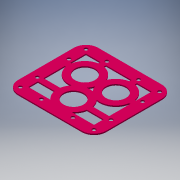
# Autodesk Inventor part: Base
Saved by Autodesk Inventor 2016 (Build 200138000, 138)
## iProperties
Created: 2015-03-29
Part Number: Base
Material: Generic
Document SubType Name: Modeling
Designer: Erin
Density: 1 g/cm^3
Appearance: Default
Author: Erin
Autodesk Inventor part; units mm, degrees
ref_plane "YZ Plane" through (0, 0, 0) normal (1, 0, 0) x (0, 1, 0)
ref_plane "XZ Plane" through (0, 0, 0) normal (0, 1, 0) x (-1, 0, 0)
ref_plane "XY Plane" through (0, 0, 0) normal (0, 0, 1) x (1, 0, 0)
sketch "Sketch1" plane through (0, 0, 0) normal (0, 0, 1) x (1, 0, 0)
  line L0 (-55, 50) -> (55, 50)
  line L1 (55, 50) -> (55, -50)
  line L2 (55, -50) -> (-55, -50)
  line L3 (-55, -50) -> (-55, 50)
  line L4 (41, 36) -> (-41, 36)
  line L5 (-41, 36) -> (-41, -36)
  line L6 (-41, -36) -> (41, -36)
  line L7 (41, -36) -> (41, 36)
  line L8 (0, 152.7233) -> (0, -72.1628) construction
  line L9 (-77.8847, 0) -> (88.8171, 0) construction
  line L10 (-55, 41) -> (55, 41) construction
  circle A0 centre (0, 41) radius 2.25
  circle A1 centre (-19.75, 41) radius 2.25
  circle A2 centre (19.75, 41) radius 2.25
  line L11 (-46, 50) -> (-46, -50) construction
  circle A3 centre (-46, 41) radius 2.25
  circle A4 centre (-46, 0) radius 2.25
  line L12 (-55, -41) -> (55, -41) construction
  circle A5 centre (-46, -41) radius 2.25
  circle A6 centre (-46, 19.75) radius 2.25
  circle A7 centre (-46, -19.75) radius 2.25
  line L13 (0, -20.5) -> (-19.3412, 13) construction
  line L14 (-19.3412, 13) -> (19.3412, 13) construction
  line L15 (19.3412, 13) -> (0, -20.5) construction
  circle A8 centre (19.3412, 13) radius 12.5
  circle A9 centre (-19.3412, 13) radius 12.5
  circle A10 centre (0, -20.5) radius 12.5
  circle A11 centre (-19.3412, 13) radius 20.5
  circle A12 centre (19.3412, 13) radius 20.5
  circle A13 centre (0, -20.5) radius 20.5
  line L16 (-22.8412, 30.0471) -> (-15.8412, 30.0471)
  line L17 (-15.8412, 30.0471) -> (-15.8412, 36)
  line L18 (-15.8412, 36) -> (-22.8412, 36)
  line L19 (-22.8412, 36) -> (-22.8412, 30.0471)
  line L20 (15.8412, 30.0471) -> (22.8412, 30.0471)
  line L21 (22.8412, 30.0471) -> (22.8412, 36)
  line L22 (22.8412, 36) -> (15.8412, 36)
  line L23 (15.8412, 36) -> (15.8412, 30.0471)
  line L24 (-35.3273, 16.5) -> (-41, 16.5)
  line L25 (-41, 16.5) -> (-41, 9.5)
  line L26 (-41, 9.5) -> (-35.3273, 9.5)
  line L27 (-35.3273, 9.5) -> (-35.3273, 16.5)
  line L28 (34.9738, 16.5) -> (41, 16.5)
  line L29 (41, 16.5) -> (41, 9.5)
  line L30 (41, 9.5) -> (34.9738, 9.5)
  line L31 (34.9738, 9.5) -> (34.9738, 16.5)
  line L32 (-3.5, -36.2367) -> (3.5, -36.2367)
  line L33 (3.5, -36.2367) -> (3.5, -36)
  line L34 (3.5, -36) -> (-3.5, -36)
  line L35 (-3.5, -36) -> (-3.5, -36.2367)
  line L36 (-16.3125, -17) -> (-41, -17)
  line L37 (-41, -17) -> (-41, -24)
  line L38 (-41, -24) -> (-16.3125, -24)
  line L39 (-16.3125, -24) -> (-16.3125, -17)
  line L40 (16.0929, -17) -> (41, -17)
  line L41 (41, -17) -> (41, -24)
  line L42 (41, -24) -> (16.0929, -24)
  line L43 (16.0929, -24) -> (16.0929, -17)
  point P0 (0, 0)
  point P1 (0, 50)
  point P2 (55, 0)
  point P3 (0, 1.8333)
  point P4 (-16.3125, -20.5)
  point P5 (16.0929, -20.5)
  point P6 (34.9738, 13)
  point P7 (-35.3273, 13)
  point P8 (-19.3412, 30.0471)
  point P9 (19.3412, 30.0471)
  point P10 (0, -36.2367)
  dimension "d0" = 110
  dimension "d1" = 100
  dimension "d2" = 14
  dimension "d5" = 9
  dimension "d6" = 4.5
  dimension "d7" = 4.5
  dimension "d8" = 4.5
  dimension "d9" = 22
  dimension "d10" = 22
  dimension "d11" = 9
  dimension "d12" = 4.5
  dimension "d13" = 4.5
  dimension "d14" = 9
  dimension "d15" = 4.5
  dimension "d31" = 4.5
  dimension "d32" = 4.5
  dimension "d33" = 22
  dimension "d34" = 22
  dimension "d53" = 23
  dimension "d54" = 25
  dimension "d55" = 25
  dimension "d56" = 25
  dimension "d65" = 8
  dimension "d66" = 8
  dimension "d67" = 8
  dimension "d68" = 7
  dimension "d69" = 7
  dimension "d70" = 7
  dimension "d71" = 7
  dimension "d72" = 7
  dimension "d73" = 7
  dimension "d74" = 7
  dimension "d75" = 38.6825
  constraints: 88 end point, 23 point on line, 19 parallel, 14 centre point, 13 perpendicular, 11 midpoint, 9 horizontal, 6 coincident, 5 horizontal alignment, 4 vertical alignment, 1 vertical, 10 other
  measures "d0" distance of L1.end L2.end
  measures "d1" distance of L0.end L1.end
  measures "d2" distance between parallel lines of L4 L0
  measures "d5" distance between parallel lines of L10 L0
  measures "d6" diameter of A0
  measures "d7" diameter of A1
  measures "d8" diameter of A2
  measures "d11" distance between parallel lines of L11 L3
  measures "d12" diameter of A3
  measures "d13" diameter of A4
  measures "d14" distance between parallel lines of L12 L2
  measures "d15" diameter of A5
  measures "d31" diameter of A6
  measures "d32" diameter of A7
  measures "d53" distance between parallel lines of L14 L4
  measures "d54" diameter of A8
  measures "d55" diameter of A9
  measures "d56" diameter of A10
  measures "d65" radial gap between concentric circles of A9 A11
  measures "d66" radial gap between concentric circles of A8 A12
  measures "d67" radial gap between concentric circles of A10 A13
  measures "d68" distance of L16.start L16.end
  measures "d69" distance of L20.start L20.end
  measures "d70" distance of L26.end L24.start
  measures "d71" distance of L30.end L28.start
  measures "d72" distance of L38.end L36.start
  measures "d73" distance of L42.end L40.start
  measures "d74" distance of L32.start L32.end
  measures "d75" distance of L13.end L14.end
extrude "Extrusion1" add sketch "Sketch1" along normal blind 1.5 contours L0 L1 L2 L3 | L21 A12 L23 L4 | L7 L30 A12 L28 | L21 L20 L23 A12 | A12 L28 L31 L30 A13 A11 L23 L20 L21 | A12 L30 L31 L28 | L17 A11 L19 L4 | L7 L42 A13 L40 | L17 L16 L19 A11 | A11 A12 A13 L26 L27 L24 L19 L16 L17 | A11 A12 | L40 L43 L42 A13 L6 L38 L39 L36 A11 A12 | A13 L42 L43 L40 | A12 A13 | L24 A11 L26 L5 | L24 L27 L26 A11 | A11 A13 | A13 L6 L35 L32 L33 | L33 L32 L35 L6 | L36 A13 L38 L5 | L36 L39 L38 A13 | A0 | A1 | A2 | A3 | A4 | A5 | A6 | A7
extrude "Extrusion2" cut sketch "Sketch1" along normal blind 10 contours A1 | A2
mirror "Mirror1" about plane through (0, 0, 0) normal (0, 1, 0) of "Extrusion2"
extrude "Extrusion3" cut sketch "Sketch1" along normal blind 10 contours A3 | A5 | A6 | A7
mirror "Mirror2" about plane through (0, 0, 0) normal (1, 0, 0) of "Extrusion3"
extrude "Extrusion7" cut sketch "Sketch1" along normal blind 10 contours L7 L28 A12 L21 L4 | L23 A12 A11 L17 L4 | L7 L40 A13 A12 L30 | L19 A11 L24 L5 L4 | L7 L6 A13 L42 | L40 L43 L42 A13 L6 L38 L39 L36 A11 A12 | A12 A13 A11 | L26 A11 A13 L36 L5 | L6 L5 L38 A13
extrude "Extrusion8" add sketch "Sketch1" along normal blind 1.5 contours L40 L43 L42 A13 L6 L38 L39 L36 A11 A12 | A13 L42 L43 L40 | A12 A13 | A11 A13 | A13 L6 L35 L32 L33 | L36 L39 L38 A13
fillet "Fillet1" radius 15 4 edges at (-55, -50, 0.75) (55, -50, 0.75) (55, 50, 0.75) (-55, 50, 0.75)
body "Solid1"
